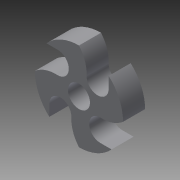
# Autodesk Inventor part: ratchet
Saved by Autodesk Inventor 2013 (Build 170138000, 138)
## iProperties
Created: 2014-01-06
Part Number: ratchet
Material: Generic
Document SubType Name: Modeling
Designer: kahohbein
Density: 1 g/cm^3
Author: kahohbein
Autodesk Inventor part; units mm, degrees
ref_plane "YZ Plane" through (0, 0, 0) normal (1, 0, 0) x (0, 1, 0)
ref_plane "XZ Plane" through (0, 0, 0) normal (0, 1, 0) x (-1, 0, 0)
ref_plane "XY Plane" through (0, 0, 0) normal (0, 0, 1) x (1, 0, 0)
sketch "Sketch1" plane through (0, 0, 0) normal (0, 0, 1) x (1, 0, 0)
  circle A0 centre (0, 0) radius 12.7
  dimension "d0" = 25.4
  constraints: 1 centre point, 1 coincident
  measures "d0" diameter of A0
extrude "Extrusion1" add sketch "Sketch1" along normal blind 6.35
sketch "Sketch2" plane through (0, 0, 6.35) normal (0, 0, 1) x (1, 0, 0)
  circle A0 centre (0, 0) radius 12.7 projected
  arc A1 (-6.4006, 2.2157) -> (-6.1091, 8.5523) centre (-6.1091, 5.3773) ccw
  line L0 (-6.1091, 8.5523) -> (-9.3887, 8.5523)
  arc A2 (-6.1091, 2.2023) -> (-12.7, 0) centre (-6.6809, -7.0502) ccw
  dimension "d3" = 6.35
  constraints: 8 point on circle, 2 centre point, 2 end point, 1 horizontal, 1 tangent
  measures "d3" diameter of A1
extrude "Extrusion2" cut sketch "Sketch2" against normal blind 50.8 contours L0 A1 A2 A0 picked at (-7.9, 5.5911)
pattern_circular "Circular Pattern1" count 4 over 360 about axis through (0, 0, -10) along (0, 0, 1) of "Extrusion2"
sketch "Sketch3" plane through (0, 0, 6.35) normal (0, 0, 1) x (1, 0, 0)
  arc A0 (12.7, 0) -> (8.5523, 9.3887) centre (0, 0) ccw projected
  circle A1 centre (0, 0) radius 3.175
  dimension "d9" = 6.35
  constraints: 1 centre point, 1 coincident
  measures "d9" diameter of A1
extrude "Extrusion3" cut sketch "Sketch3" against normal blind 50.8
body "Solid1"
